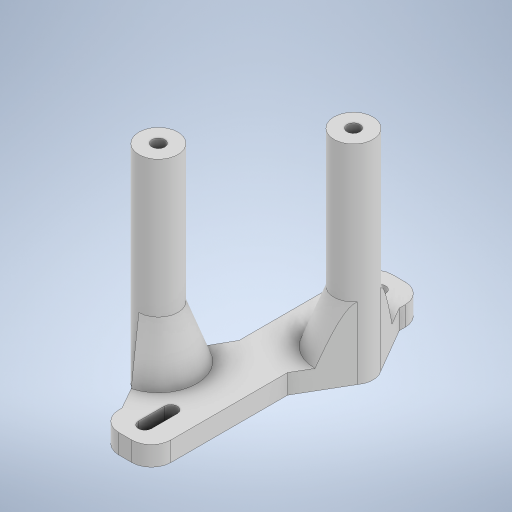
# Autodesk Inventor part: supporto_mb1202
Saved by Autodesk Inventor 2023.2 (Build 272271030, 271C)
## iProperties
Created: 2023-11-07
Part Number: supporto_mb1202
Material: Generic
Document SubType Name: Modeling
Designer: matti
Density: 1 g/cm^3
Appearance: Default
Author: matti
Autodesk Inventor part; units mm, degrees
ref_plane "YZ Plane" through (0, 0, 0) normal (1, 0, 0) x (0, 1, 0)
ref_plane "XZ Plane" through (0, 0, 0) normal (0, 1, 0) x (-1, 0, 0)
ref_plane "XY Plane" through (0, 0, 0) normal (0, 0, 1) x (1, 0, 0)
sketch "Sketch1" plane through (0, 0, 0) normal (0, 1, 0) x (-1, 0, 0)
  arc A0 (-1, 14) -> (1, 14) centre (0, 14) ccw
  line L0 (0, -43.0187) -> (0, 32.3947) projected
  arc A1 (1, 18) -> (-1, 18) centre (0, 18) ccw
  line L1 (1, 18) -> (1, 14)
  line L2 (-1, 14) -> (-1, 18)
  line L3 (0, 18) -> (0, 16)
  line L4 (3.8037, 16) -> (0, 16) construction
  line L5 (14.482, 0) -> (-14.022, 0) construction
  arc A2 (1, -14) -> (-1, -14) centre (0, -14) ccw
  arc A3 (-1, -18) -> (1, -18) centre (0, -18) ccw
  line L6 (1, -18) -> (1, -14)
  line L7 (-1, -14) -> (-1, -18)
  line L8 (3.8037, -16) -> (0, -16) construction
  line L9 (1, 21) -> (-1, 21)
  line L10 (-4, 18) -> (-4, -18)
  line L11 (-1, -21) -> (1, -21)
  line L12 (4, -18) -> (4, 18)
  arc A4 (4, 18) -> (1, 21) centre (1, 18) ccw
  arc A5 (-1, 21) -> (-4, 18) centre (-1, 18) ccw
  arc A6 (-4, -18) -> (-1, -21) centre (-1, -18) ccw
  arc A7 (1, -21) -> (4, -18) centre (1, -18) ccw
  line L13 (9.95, -10.51) -> (-9.95, -10.51) construction
  line L14 (-9.95, -10.51) -> (-9.95, 10.51) construction
  line L15 (9.95, 10.51) -> (9.95, -10.51) construction
  circle A8 centre (7.41, 8.51) radius 1
  circle A9 centre (-5.55, -8.49) radius 0.75 construction
  line L16 (0, -32.2454) -> (0, -10.51) construction
  line L17 (9.95, 0) -> (-9.95, 0) construction
  line L18 (9.95, 10.51) -> (-9.95, 10.51) construction
  line L19 (4, 10.51) -> (9, 10.51) construction
  line L20 (9, 10.51) -> (9, 6.51) construction
  line L21 (9, 6.51) -> (4, 6.51) construction
  line L22 (4, 6.51) -> (4, 10.51)
  line L23 (7.41, 8.51) -> (9.1387, 8.51) construction
  circle A10 centre (7.41, 8.51) radius 3
  line L24 (7.41, 11.51) -> (4, 11.51)
  line L25 (7.41, 5.51) -> (4, 5.51)
  arc A11 (-4, -7.2261) -> (-4, -9.7539) centre (-5.55, -8.49) ccw construction
  line L26 (-5.55, -6.49) -> (-4, -6.49) construction
  line L27 (-5.55, -10.49) -> (-4, -10.49) construction
  circle A12 centre (-5.55, -8.49) radius 2 construction
  line L28 (-7.55, -8.49) -> (-7.55, -26.4012) construction
  circle A13 centre (-5.55, -8.49) radius 3
  circle A14 centre (-5.55, -8.49) radius 1
  point P0 (0, 0)
  point P1 (0, 21)
  point P2 (0, 19)
  point P3 (-5.55, -6.94)
  point P4 (-4, -6.94)
  point P5 (-5.55, -10.04)
  point P6 (-4, -10.04)
  point P7 (4, 5.51)
  point P8 (4, 11.51)
  point P9 (-4, -9.7539)
  point P10 (-4, -9.7539)
  dimension "d4" = 2
  dimension "d7" = 2
  dimension "d14" = 2
  dimension "d15" = 16
  dimension "d16" = 2
  dimension "d17" = 2
  dimension "d18" = 16
  dimension "d19" = 42
  dimension "d21" = 8
  dimension "d22" = 3
  dimension "d24" = 19.9
  dimension "d31" = 2.54
  dimension "d33" = 17
  dimension "d34" = 19.9
  dimension "d36" = 15.5
  dimension "d37" = 5
  dimension "d38" = 4
  dimension "d39" = 2
  dimension "d40" = 1.5
  dimension "d45" = 4
  dimension "d46" = 6
  dimension "d51" = 7.55
  dimension "d64" = 6
  dimension "d65" = 2
  constraints: 54 end point, 24 point on circle, 16 tangent, 14 centre point, 11 point on line, 8 symmetric about line, 7 perpendicular, 5 parallel, 4 coincident, 4 midpoint, 3 equal radius, 3 horizontal, 2 collinear, 1 vertical, 9 other
  measures "d4" diameter of A0
  measures "d7" diameter of A1
  measures "d14" distance from line of L3.start L4
  measures "d15" distance between parallel lines of L5 L4
  measures "d16" distance of A0.centre L3.end
  measures "d17" distance of L3.start L3.end
  measures "d18" distance between parallel lines of L5 L8
  measures "d19" distance between parallel lines of L11 L9
  measures "d21" distance between parallel lines of L10 L12
  measures "d22" radius of A4
  measures "d24" distance of L14.end L15.start
  measures "d31" distance from line of L15 L23.start
  measures "d33" vertical distance of A9.centre L23.start
  measures "d34" distance between parallel lines of L14 L15
  measures "d36" distance from line of A9.centre L15
  measures "d37" distance of L20.end L21.end
  measures "d38" distance of L19.end L20.end
  measures "d39" diameter of A8
  measures "d40" diameter of A9
  measures "d45" diameter of A11
  measures "d46" diameter of A10
  measures "d51" distance between parallel lines of L28 L0
  measures "d64" diameter of A13
  measures "d65" diameter of A14
extrude "Extrusion2" add sketch "Sketch1" along normal blind 32 contours A10 | A8
extrude "Extrusion3" add sketch "Sketch1" along normal blind 32 contours A13 L10 | L10 A13 | A14
extrude "Extrusion4" add sketch "Sketch1" along normal blind 3 contours A0 L0 A2 L7 A3 L11 A6 L10 A13 A5 L9 A1 L2 | A0 L1 A1 L0 L9 A4 L12 A7 L11 A3 L6 A2 | L24 A10 L25 L12 | A13 L10 picked at (-3.0537, -8.3357)
chamfer "Chamfer1" distance 4 distance2 6 2 edges at (4, 1.5, -11.0586) (4, 1.5, -5.9214) measured on face at (8.55, 10.6667, -8.49)
chamfer_without_effect "Chamfer2"
chamfer "Chamfer3" distance 6 distance2 3.4 1 edges at (-4, 1.5, 5.51) measured on face at (-4, 1, -10.1633)
chamfer "Chamfer4" distance 3.4 distance2 6 1 edges at (-4, 1.5, 11.51) measured on face at (-6.2733, 1, 11.51)
chamfer "Chamfer5" distance 8 angle 20 1 edges at (-4.41, 3, 8.51)
chamfer "Chamfer6" distance 8 angle 20 2 edges at (4.586, 3, -5.6491) (4.586, 3, -11.3309) measured on face at (8.3281, 21.3333, -9.6224)
sketch "Sketch2" plane through (-7.41, 32, 8.51) normal (0, 1, 0) x (1, 0, 0)
  circle A0 centre (0, 0) radius 3 projected
  circle A1 centre (0, 0) radius 1
  circle A2 centre (12.96, 17) radius 3 projected
  circle A3 centre (12.96, 17) radius 1
  point P0 (7.41, 8.51)
  dimension "d72" = 2
  dimension "d73" = 2
  constraints: 2 centre point, 2 coincident
  measures "d72" diameter of A1
  measures "d73" diameter of A3
extrude "Extrusion5" cut sketch "Sketch2" against normal blind 8 contours A1 | A3
body "Solid1"
